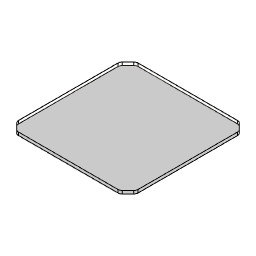
Front Transparent-T1 v5 (Autodesk Fusion 360 design; units mm, degrees)
Autodesk Fusion 360 part; units mm, degrees
sketch "Sketch1" plane through (0, 0, 0) normal (0, 1, 0) x (1, 0, 0)
  line L0 (57.9284, 52.2684) -> (52.2684, 57.9284)
  arc A0 (52.2684, 57.9284) -> (49.44, 59.1) centre (49.44, 55.1) ccw
  line L1 (49.44, 59.1) -> (-49.44, 59.1)
  arc A1 (-49.44, 59.1) -> (-52.2684, 57.9284) centre (-49.44, 55.1) ccw
  line L2 (-52.2684, 57.9284) -> (-57.9284, 52.2684)
  arc A2 (-57.9284, 52.2684) -> (-59.1, 49.44) centre (-55.1, 49.44) ccw
  line L3 (-59.1, 49.44) -> (-59.1, -49.44)
  arc A3 (-59.1, -49.44) -> (-57.9284, -52.2684) centre (-55.1, -49.44) ccw
  line L4 (-57.9284, -52.2684) -> (-52.2684, -57.9284)
  arc A4 (-52.2684, -57.9284) -> (-49.44, -59.1) centre (-49.44, -55.1) ccw
  line L5 (-49.44, -59.1) -> (49.44, -59.1)
  arc A5 (49.44, -59.1) -> (52.2684, -57.9284) centre (49.44, -55.1) ccw
  line L6 (52.2684, -57.9284) -> (57.9284, -52.2684)
  arc A6 (57.9284, -52.2684) -> (59.1, -49.44) centre (55.1, -49.44) ccw
  line L7 (59.1, -49.44) -> (59.1, 49.44)
  arc A7 (59.1, 49.44) -> (57.9284, 52.2684) centre (55.1, 49.44) ccw
  line L8 (-57.2213, -51.5613) -> (-51.5613, -57.2213)
  arc A8 (-51.5613, -57.2213) -> (-49.44, -58.1) centre (-49.44, -55.1) ccw
  line L9 (-49.44, -58.1) -> (49.44, -58.1)
  arc A9 (49.44, -58.1) -> (51.5613, -57.2213) centre (49.44, -55.1) ccw
  line L10 (51.5613, -57.2213) -> (57.2213, -51.5613)
  arc A10 (57.2213, -51.5613) -> (58.1, -49.44) centre (55.1, -49.44) ccw
  line L11 (58.1, -49.44) -> (58.1, 49.44)
  arc A11 (58.1, 49.44) -> (57.2213, 51.5613) centre (55.1, 49.44) ccw
  line L12 (57.2213, 51.5613) -> (51.5613, 57.2213)
  arc A12 (51.5613, 57.2213) -> (49.44, 58.1) centre (49.44, 55.1) ccw
  line L13 (49.44, 58.1) -> (-49.44, 58.1)
  arc A13 (-49.44, 58.1) -> (-51.5613, 57.2213) centre (-49.44, 55.1) ccw
  line L14 (-51.5613, 57.2213) -> (-57.2213, 51.5613)
  arc A14 (-57.2213, 51.5613) -> (-58.1, 49.44) centre (-55.1, 49.44) ccw
  line L15 (-58.1, 49.44) -> (-58.1, -49.44)
  arc A15 (-58.1, -49.44) -> (-57.2213, -51.5613) centre (-55.1, -49.44) ccw
  line L16 (-59.1, 35) -> (59.1, 35)
  line L17 (59.1, 35) -> (59.1, 25)
  line L18 (59.1, 25) -> (-59.1, 25)
  line L19 (-59.1, 25) -> (-59.1, 35)
  line L20 (-59.1, -25) -> (59.1, -25)
  line L21 (59.1, -25) -> (59.1, -35)
  line L22 (59.1, -35) -> (-59.1, -35)
  line L23 (-59.1, -35) -> (-59.1, -25)
  line L24 (-35, 59.1) -> (-25, 59.1)
  line L25 (-25, 59.1) -> (-25, -59.1)
  line L26 (-25, -59.1) -> (-35, -59.1)
  line L27 (-35, -59.1) -> (-35, 59.1)
  line L28 (25, 59.1) -> (35, 59.1)
  line L29 (35, 59.1) -> (35, -59.1)
  line L30 (35, -59.1) -> (25, -59.1)
  line L31 (25, -59.1) -> (25, 59.1)
  line L32 (58.777, 53.117) -> (53.117, 58.777)
  arc A16 (53.117, 58.777) -> (49.44, 60.3) centre (49.44, 55.1) ccw
  line L33 (49.44, 60.3) -> (-49.44, 60.3)
  arc A17 (-49.44, 60.3) -> (-53.117, 58.777) centre (-49.44, 55.1) ccw
  line L34 (-53.117, 58.777) -> (-58.777, 53.117)
  arc A18 (-58.777, 53.117) -> (-60.3, 49.44) centre (-55.1, 49.44) ccw
  line L35 (-60.3, 49.44) -> (-60.3, -49.44)
  arc A19 (-60.3, -49.44) -> (-58.777, -53.117) centre (-55.1, -49.44) ccw
  line L36 (-58.777, -53.117) -> (-53.117, -58.777)
  arc A20 (-53.117, -58.777) -> (-49.44, -60.3) centre (-49.44, -55.1) ccw
  line L37 (-49.44, -60.3) -> (49.44, -60.3)
  arc A21 (49.44, -60.3) -> (53.117, -58.777) centre (49.44, -55.1) ccw
  line L38 (53.117, -58.777) -> (58.777, -53.117)
  arc A22 (58.777, -53.117) -> (60.3, -49.44) centre (55.1, -49.44) ccw
  line L39 (60.3, -49.44) -> (60.3, 49.44)
  arc A23 (60.3, 49.44) -> (58.777, 53.117) centre (55.1, 49.44) ccw
  line L40 (58.1406, 52.4806) -> (52.4806, 58.1406)
  arc A24 (52.4806, 58.1406) -> (49.44, 59.4) centre (49.44, 55.1) ccw
  line L41 (49.44, 59.4) -> (-49.44, 59.4)
  arc A25 (-49.44, 59.4) -> (-52.4806, 58.1406) centre (-49.44, 55.1) ccw
  line L42 (-52.4806, 58.1406) -> (-58.1406, 52.4806)
  arc A26 (-58.1406, 52.4806) -> (-59.4, 49.44) centre (-55.1, 49.44) ccw
  line L43 (-59.4, 49.44) -> (-59.4, -49.44)
  arc A27 (-59.4, -49.44) -> (-58.1406, -52.4806) centre (-55.1, -49.44) ccw
  line L44 (-58.1406, -52.4806) -> (-52.4806, -58.1406)
  arc A28 (-52.4806, -58.1406) -> (-49.44, -59.4) centre (-49.44, -55.1) ccw
  line L45 (-49.44, -59.4) -> (49.44, -59.4)
  arc A29 (49.44, -59.4) -> (52.4806, -58.1406) centre (49.44, -55.1) ccw
  line L46 (52.4806, -58.1406) -> (58.1406, -52.4806)
  arc A30 (58.1406, -52.4806) -> (59.4, -49.44) centre (55.1, -49.44) ccw
  line L47 (59.4, -49.44) -> (59.4, 49.44)
  arc A31 (59.4, 49.44) -> (58.1406, 52.4806) centre (55.1, 49.44) ccw
  dimension "d27" = 118.2
  dimension "d28" = 118.2
  dimension "d29" = 59.1
  dimension "d30" = 59.1
  dimension "d31" = 4
  dimension "d32" = 4
  dimension "d33" = 4
  dimension "d34" = 4
  dimension "d35" = 9.66
  dimension "d36" = 9.66
  dimension "d37" = 9.66
  dimension "d38" = 9.66
  dimension "d39" = 4
  dimension "d40" = 4
  dimension "d41" = 4
  dimension "d42" = 4
  dimension "d43" = 9.66
  dimension "d44" = 9.66
  dimension "d45" = 9.66
  dimension "d46" = 9.66
  dimension "d47" = -1
  dimension "d48" = 50
  dimension "d49" = 25
  dimension "d50" = 10
  dimension "d51" = 10
  dimension "d52" = 50
  dimension "d53" = 10
  dimension "d54" = 10
  dimension "d55" = 25
  dimension "d59" = 1.2
  dimension "d60" = 120.6
  dimension "d61" = 0.3
  constraint tangent L0 A7
  constraint tangent L0 A0
  constraint tangent A0 L1
  constraint tangent A5 L6
  constraint tangent L1 A1
  constraint tangent L3 A3
  constraint tangent A1 L2
  constraint tangent L2 A2
  constraint tangent L5 A5
  constraint tangent A2 L3
  constraint tangent A3 L4
  constraint tangent L4 A4
  constraint tangent A4 L5
  constraint tangent L6 A6
  constraint tangent A6 L7
  constraint tangent L7 A7
  constraint horizontal L5
  constraint vertical L3
  constraint horizontal L16
  constraint vertical L17
  constraint horizontal L18
  constraint vertical L19
  constraint coincident L7 L17.end
  constraint coincident L3 L16.start
  constraint horizontal L20
  constraint vertical L21
  constraint horizontal L22
  constraint vertical L23
  constraint coincident L7 L21.end
  constraint coincident L3 L20.start
  constraint horizontal L24
  constraint vertical L25
  constraint horizontal L26
  constraint vertical L27
  constraint coincident L5 L25.end
  constraint coincident L1 L24.start
  constraint horizontal L28
  constraint vertical L29
  constraint horizontal L30
  constraint vertical L31
  constraint coincident L1 L28.start
  measures "d27" distance of L1 L5
  measures "d28" distance of L3 L7
  measures "d29" distance of origin L7
  measures "d30" distance of origin L5
  measures "d31" radius of A4
  measures "d32" radius of A3
  measures "d33" radius of A5
  measures "d34" radius of A6
  measures "d35" distance of A5.centre L7
  measures "d36" distance of L5 A6.centre
  measures "d37" distance of L3 A4.centre
  measures "d38" distance of A3.centre L5
  measures "d39" radius of A2
  measures "d40" radius of A1
  measures "d41" radius of A0
  measures "d42" radius of A7
  measures "d43" distance of L1 A7.centre
  measures "d44" distance of A0.centre L7
  measures "d45" distance of A1.centre L3
  measures "d46" distance of L1 A2.centre
  measures "d48" distance of L18 L20
  measures "d49" distance of origin L18
  measures "d50" distance of L16 L18
  measures "d51" distance of L20 L22
  measures "d52" distance of L25 L31
  measures "d53" distance of L29 L31
  measures "d54" distance of L25 L27
  measures "d55" distance of origin L31
  measures "d60" distance of L35 L39
extrude "Extrude1" add sketch "Sketch1" against normal blind 3 contours L0 A0 L1 L7 A7 L11 A11 L12 A12 L13 L16 L29 | L7 L11 L16 L17 L18 | L1 L13 L28 L29 L31 | L7 L11 L18 L20 | L11 A11 L12 A12 L13 L16 L29 | L11 L16 L18 L29 | L1 L13 L25 L31 | L13 L16 L29 L31 | L7 L11 L20 L21 L22 | L11 L18 L20 L29 | L16 L18 L29 L31 | L1 L13 L24 L25 L27 | L13 L16 L25 L31 | L5 A5 L6 A6 L7 L9 A9 L10 A10 L11 L22 L29 | L11 L20 L22 L29 | L18 L20 L29 L31 | L16 L18 L25 L31 | L1 A1 L2 A2 L3 L13 A13 L14 A14 L15 L16 L27 | L13 L16 L25 L27 | L9 A9 L10 A10 L11 L22 L29 | L20 L22 L29 L31 | L18 L20 L25 L31 | L16 L18 L25 L27 | L13 A13 L14 A14 L15 L16 L27 | L9 L22 L29 L31 | L20 L22 L25 L31 | L18 L20 L25 L27 | L15 L16 L18 L27 | L9 L22 L25 L31 | L5 L9 L29 L30 L31 | L20 L22 L25 L27 | L15 L18 L20 L27 | L3 L15 L16 L18 L19 | L9 L22 L25 L27 | L5 L9 L25 L31 | L15 L20 L22 L27 | L3 L15 L18 L20 | L8 A8 L9 L15 A15 L22 L27 | L5 L9 L25 L26 L27 | L3 L15 L20 L22 L23 | L3 A3 L4 A4 L5 L8 A8 L9 L15 A15 L22 L27 | L40 A24 L41 A25 L42 A26 L43 A27 L44 A28 L45 A29 L46 A30 L47 A31
equation "d29 = d28 / 2"
equation "d30 = d27 / 2"
equation "d49 = d48 / 2"
equation "d55 = d52 / 2"
